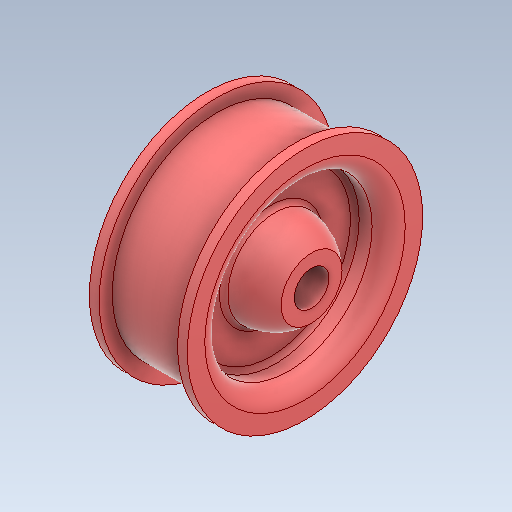
# Autodesk Inventor part: Wheel 75 mm - Part 2
Saved by Autodesk Inventor 2020 (Build 240168000, 168)
## iProperties
Created: 2023-01-26
Part Number: Wheel 75 mm - Part 2
Material: Polypropylene
Document SubType Name: Modeling
Designer: saad.nashed
Density: 0.899 g/cm^3
Appearance: Smooth - Red
d12: 4.000 mm
d17: 25.500 mm
Author: saad.nashed
Autodesk Inventor part; units mm, degrees
ref_plane "YZ Plane" through (0, 0, 0) normal (1, 0, 0) x (0, 1, 0)
ref_plane "XZ Plane" through (0, 0, 0) normal (0, 1, 0) x (-1, 0, 0)
ref_plane "XY Plane" through (0, 0, 0) normal (0, 0, 1) x (1, 0, 0)
sketch "Sketch1" plane through (0, 0, 0) normal (0, 1, 0) x (-1, 0, 0)
  line L0 (11.25, -27) -> (9, -27)
  line L1 (9, -27) -> (9, -24)
  line L2 (9, -24) -> (-9, -24)
  line L3 (-9, -24) -> (-9, -27)
  line L4 (-9, -27) -> (-11.25, -27)
  line L5 (-11.25, -27) -> (-11.25, -23)
  arc A0 (-7.45, -19.2) -> (-11.25, -23) centre (-7.45, -23) ccw
  line L6 (-7.45, -19.2) -> (-4.48, -19.2)
  line L7 (-3.48, -18.2) -> (-3.48, -11.8672)
  line L8 (0, 0) -> (0, -6.0117) construction
  line L9 (0, 0) -> (7.1191, 0) construction
  line L10 (11.25, -27) -> (11.25, -23)
  arc A1 (11.25, -23) -> (7.45, -19.2) centre (7.45, -23) ccw
  line L11 (7.45, -19.2) -> (4.48, -19.2)
  line L12 (3.48, -18.2) -> (3.48, -11.8672)
  arc A2 (4.4084, -10.8697) -> (12.75, -7) centre (3.48, 2.057) ccw
  line L13 (12.75, -7) -> (12.75, -4)
  line L14 (12.75, -4) -> (-12.75, -4)
  arc A3 (-12.75, -7) -> (-4.4084, -10.8697) centre (-3.48, 2.057) ccw
  line L15 (-12.75, -7) -> (-12.75, -4)
  arc A4 (4.4084, -10.8697) -> (3.48, -11.8672) centre (4.48, -11.8672) ccw
  arc A5 (3.48, -18.2) -> (4.48, -19.2) centre (4.48, -18.2) ccw
  arc A6 (-3.48, -11.8672) -> (-4.4084, -10.8697) centre (-4.48, -11.8672) ccw
  arc A7 (-4.48, -19.2) -> (-3.48, -18.2) centre (-4.48, -18.2) ccw
  point P0 (-3.48, -19.2)
  point P1 (-3.48, -10.903)
  point P2 (3.48, -19.2)
  point P3 (3.48, -10.903)
  dimension "d0" = 22.5
  dimension "d2" = 2.25
  dimension "d6" = 3
  dimension "d7" = 24
  dimension "d8" = 4.8
  dimension "d9" = 3.8
  dimension "d10" = 6.96
  dimension "d11" = 12.96
  dimension "d12" = 4
  dimension "d13" = 3
  dimension "d15" = 1.5
  dimension "d16" = 1
  dimension "d17" = 25.5
  constraints: 32 end point, 18 point on circle, 11 tangent, 9 point on line, 8 centre point, 6 perpendicular, 4 horizontal, 4 symmetric about line, 3 equal radius, 3 vertical, 1 parallel, 7 other
  measures "d0" distance between parallel lines of L5 L10
  measures "d2" distance between parallel lines of L1 L10
  measures "d6" distance between parallel lines of L0 L2
  measures "d7" distance between parallel lines of L9 L2
  measures "d8" distance between parallel lines of L2 L6
  measures "d9" radius of A0
  measures "d10" distance between parallel lines of L7 L12
  measures "d11" radius of A2
  measures "d12" distance between parallel lines of L14 L9
  measures "d13" distance from line of L13.start L14
  measures "d15" distance between parallel lines of L5 L15
  measures "d16" radius of A4
  measures "d17" distance between parallel lines of L15 L13
revolve "Revolution1" add sketch "Sketch1" angle 360 about axis through (0, 0, 0) along (-1, 0, 0)
equation "\"d0\" = d1 + 2 * d5"
equation "\"d2\" = 2 * d5"
equation "\"d6\" = d4"
equation "\"d7\" = d3"
equation "\"d8\" = 0.2 * d7"
equation "\"d10\" = 0.29 * d7"
equation "\"d11\" = 0.54 * d7"
equation "\"d13\" = d6"
equation "\"d1\" = 20.25"
equation "\"d5\" = 1.125"
equation "\"d4\" = 3"
equation "\"d3\" = 24"
body "Solid1"
